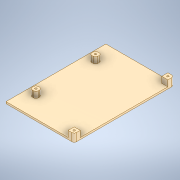
# Autodesk Inventor part: VIM1_Holder
Saved by Autodesk Inventor 2020 (Build 240168000, 168)
## iProperties
Created: 2020-04-26
Part Number: VIM1_Holder
Material: Типовые
Document SubType Name: Modeling
Designer: Михаил
Density: 1 g/cm^3
Appearance: По умолчанию
Author: Михаил
Autodesk Inventor part; units mm, degrees
ref_plane "YZ Plane" through (0, 0, 0) normal (1, 0, 0) x (0, 1, 0)
ref_plane "XZ Plane" through (0, 0, 0) normal (0, 1, 0) x (-1, 0, 0)
ref_plane "XY Plane" through (0, 0, 0) normal (0, 0, 1) x (1, 0, 0)
sketch "Эскиз1" plane through (0, 0, 0) normal (0, 1, 0) x (-1, 0, 0)
  line L0 (0, 0) -> (56, 0)
  line L1 (56, 0) -> (56, -82)
  line L2 (56, -82) -> (0, -82)
  line L3 (0, -82) -> (0, 0)
  dimension "d0" = 56
  dimension "d1" = 82
  constraints: 8 end point, 2 parallel, 1 horizontal, 1 perpendicular
  measures "d0" distance of L1.end L2.end
  measures "d1" distance of L0.end L1.end
extrude "Выдавливание1" add sketch "Эскиз1" along normal blind 1.5
sketch "Эскиз2" plane through (0, 1.5, 0) normal (0, 1, 0) x (1, 0, 0)
  line L0 (-56, 0) -> (0, 0) projected
  line L1 (0, 0) -> (-5, 0)
  line L2 (-5, 0) -> (-5, 5)
  line L3 (-5, 5) -> (0, 5)
  line L4 (0, 5) -> (0, 0)
  line L5 (0, 0) -> (0, 82) projected
  line L6 (0, 82) -> (-5, 82)
  line L7 (-5, 82) -> (-5, 77)
  line L8 (-5, 77) -> (0, 77)
  line L9 (0, 77) -> (0, 82)
  line L10 (-50.5, 14) -> (-45.5, 14)
  line L11 (-45.5, 14) -> (-45.5, 19)
  line L12 (-45.5, 19) -> (-50.5, 19)
  line L13 (-50.5, 19) -> (-50.5, 14)
  line L14 (-50.5, 63) -> (-45.5, 63)
  line L15 (-45.5, 63) -> (-45.5, 68)
  line L16 (-45.5, 68) -> (-50.5, 68)
  line L17 (-50.5, 68) -> (-50.5, 63)
  line L18 (-56, 82) -> (-56, 0) projected
  line L19 (0, 82) -> (-56, 82) projected
  dimension "d4" = 5
  dimension "d5" = 5
  dimension "d6" = 5
  dimension "d7" = 5
  dimension "d8" = 5
  dimension "d9" = 5
  dimension "d10" = 5
  dimension "d11" = 5
  dimension "d12" = 14
  dimension "d13" = 5.5
  dimension "d14" = 14
  constraints: 32 end point, 8 parallel, 4 horizontal, 4 perpendicular, 1 point on line
  measures "d4" distance of L2.end L3.end
  measures "d5" distance of L1.end L2.end
  measures "d6" distance of L8.end L7.end
  measures "d7" distance of L7.end L6.end
  measures "d8" distance of L12.end L11.end
  measures "d9" distance of L11.end L10.end
  measures "d10" distance of L16.end L15.end
  measures "d11" distance of L15.end L14.end
  measures "d12" distance between parallel lines of L0 L10
  measures "d13" distance between parallel lines of L18 L13
  measures "d14" distance between parallel lines of L19 L16
extrude "Выдавливание2" add sketch "Эскиз2" along normal blind 5 contours L2 L3 L4 L0 | L6 L5 L8 L7 | L13 L12 L11 L10 | L17 L16 L15 L14
sketch "Эскиз3" plane through (0, 6.5, 0) normal (0, 1, 0) x (1, 0, 0)
  circle A0 centre (-2.5, 2.5) radius 0.75
  line L0 (-5, 0) -> (0, 0) projected
  line L1 (0, 0) -> (0, 5) projected
  circle A1 centre (-2.5, 79.5) radius 0.75
  line L2 (0, 77) -> (0, 82) projected
  line L3 (0, 82) -> (-5, 82) projected
  circle A2 centre (-48, 16.5) radius 0.75
  line L4 (-56, 0) -> (-5, 0) projected
  circle A3 centre (-48, 65.5) radius 0.75
  line L5 (-5, 82) -> (-56, 82) projected
  line L6 (-45.5, 14) -> (-45.5, 19) projected
  line L7 (-45.5, 63) -> (-45.5, 68) projected
  dimension "d17" = 1.5
  dimension "d18" = 2.5
  dimension "d19" = 2.5
  dimension "d20" = 1.5
  dimension "d21" = 2.5
  dimension "d22" = 2.5
  dimension "d23" = 1.5
  dimension "d24" = 16.5
  dimension "d25" = 1.5
  dimension "d26" = 16.5
  dimension "d27" = 2.5
  dimension "d28" = 2.5
  constraints: 4 centre point
  measures "d17" diameter of A0
  measures "d18" distance from line of L0 A0.centre
  measures "d19" distance from line of L1 A0.centre
  measures "d20" diameter of A1
  measures "d21" distance from line of L2 A1.centre
  measures "d22" distance from line of L3 A1.centre
  measures "d23" diameter of A2
  measures "d24" distance from line of L4 A2.centre
  measures "d25" diameter of A3
  measures "d26" distance from line of L5 A3.centre
  measures "d27" distance from line of L6 A2.centre
  measures "d28" distance from line of L7 A3.centre
extrude "Выдавливание3" cut sketch "Эскиз3" against normal blind 5
fillet "Сопряжение1" radius 2 10 edges at (0, 3.25, 0) (0, 3.25, -82) (-45.5, 4, -14) (-45.5, 4, -19) (-50.5, 4, -14) (-50.5, 4, -19) (-45.5, 4, -63) (-45.5, 4, -68) (-50.5, 4, -68) (-50.5, 4, -63)
